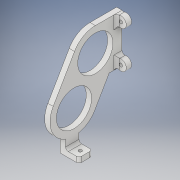
# Autodesk Inventor part: Tank Mount
Saved by Autodesk Inventor 2019.4 (Build 234330000, 330)
## iProperties
Created: 2020-01-30
Part Number: Tank Mount
Material: ABS Plastic
Document SubType Name: Modeling
Designer: admin
Mass: 80 g
Surface Area: 347.05 cm^2
Volume: 116.718 cm^3
Density: 0.685414 g/cm^3
Appearance: Smooth - White
Author: admin
Autodesk Inventor part; units mm, degrees
ref_plane "YZ Plane" through (0, 0, 0) normal (1, 0, 0) x (0, 1, 0)
ref_plane "XZ Plane" through (0, 0, 0) normal (0, 1, 0) x (-1, 0, 0)
ref_plane "XY Plane" through (0, 0, 0) normal (0, 0, 1) x (1, 0, 0)
sketch "Sketch1" plane through (0, 0, 0) normal (1, 0, 0) x (0, 1, 0)
  circle A0 centre (0, 0) radius 33
  circle A1 centre (69.282, -40) radius 33
  line L0 (0, 0) -> (69.282, -40) construction
  line L1 (69.282, -40) -> (69.282, -90) construction
  arc A2 (91.782, -1.0289) -> (114.282, -40) centre (69.282, -40) ccw construction
  arc A3 (-42.1724, 15.7) -> (-44.0285, -9.3) centre (0, 0) ccw construction
  line L2 (22.5, 38.9711) -> (91.782, -1.0289)
  line L3 (46.782, -78.9711) -> (24.282, -65.9808) construction
  line L4 (114.282, -40) -> (114.282, -90)
  line L5 (114.282, -90) -> (24.282, -90)
  line L6 (24.282, -90) -> (24.282, -65.9808)
  arc A4 (114.282, -40) -> (91.782, -1.0289) centre (69.282, -40) ccw
  line L7 (-70, 15.7) -> (-70, -9.3)
  line L8 (-70, 15.7) -> (-42.1724, 15.7)
  line L9 (-70, -9.3) -> (-44.0285, -9.3)
  arc A5 (22.5, 38.9711) -> (-42.1724, 15.7) centre (0, 0) ccw
  line L10 (24.282, -65.9808) -> (24.282, -40) construction
  line L11 (24.282, -65.9808) -> (-22.5, -38.9711)
  arc A6 (-22.5, -38.9711) -> (22.5, 38.9711) centre (0, 0) ccw construction
  arc A7 (-44.0285, -9.3) -> (-22.5, -38.9711) centre (0, 0) ccw
  dimension "d0" = 66
  dimension "d1" = 66
  dimension "d2" = 80
  dimension "d3" = 50
  dimension "d4" = 90
  dimension "d5" = 90
  dimension "d6" = 90
  dimension "d7" = 50
  dimension "d8" = 25
  dimension "d9" = 70
  dimension "d10" = 105.7
  constraints: 24 end point, 15 point on circle, 13 tangent, 8 centre point, 3 coincident, 3 parallel, 3 perpendicular, 3 vertical, 1 horizontal
  measures "d0" diameter of A0
  measures "d1" diameter of A1
  measures "d2" distance of L0.start L0.end
  measures "d3" distance of L0.end L1.end
  measures "d4" vertical distance of L1.end L0.start
  measures "d5" diameter of A2
  measures "d6" diameter of A3
  measures "d7" distance of L4.start L4.end
  measures "d8" distance of L7.start L7.end
  measures "d9" distance from line of point (0, 0) L7
  measures "d10" distance between parallel lines of L5 L8
extrude "Extrusion1" add sketch "Sketch1" along normal blind 10
sketch "Sketch2" plane through (0, -70, -9.3) normal (0, -1, 0) x (1, 0, 0)
  line L0 (0, 25) -> (35, 25)
  line L1 (35, 25) -> (35, 0)
  line L2 (35, 0) -> (0, 0)
  line L3 (0, 0) -> (0, 25)
  line L4 (0, 0) -> (0, 25) projected
  line L5 (0, 0) -> (10, 0) projected
  line L6 (10, 25) -> (10, 0) projected
  line L7 (0, 25) -> (10, 25) projected
  line L8 (0, 25) -> (10, 25) projected
  circle A0 centre (25, 12.5) radius 3
  line L9 (0, 48.2711) -> (0, 8.2711) projected
  point P0 (0, 9.3)
  dimension "d13" = 6
  dimension "d17" = 10
  dimension "d31" = 25
  constraints: 8 end point, 3 collinear, 2 parallel, 1 centre point, 1 horizontal, 1 perpendicular
  measures "d13" diameter of A0
  measures "d17" distance from line of L1 A0.centre
  measures "d31" distance between parallel lines of L6 L1
extrude "Extrusion2" add sketch "Sketch2" against normal blind 10 contours L0 L1 L2 L6
sketch "Sketch3" plane through (0, 24.282, -90) normal (0, 0, -1) x (-1, 0, 0)
  circle A0 centre (-18, 80) radius 3
  circle A1 centre (-18, 80) radius 10
  circle A2 centre (-18, 10) radius 3
  circle A3 centre (-18, 10) radius 10
  line L0 (0, 0) -> (-10, 0) projected
  line L1 (0, 90) -> (-10, 90) projected
  line L2 (0, 90) -> (0, 0) projected
  point P0 (0, -24.282)
  dimension "d23" = 6
  dimension "d24" = 20
  dimension "d25" = 6
  dimension "d26" = 20
  dimension "d32" = 18
  dimension "d33" = 18
  dimension "d36" = 10
  dimension "d37" = 10
  constraints: 4 centre point, 2 coincident
  measures "d23" diameter of A0
  measures "d24" diameter of A1
  measures "d25" diameter of A2
  measures "d26" diameter of A3
  measures "d32" distance from line of L2 A1.centre
  measures "d33" distance from line of L2 A3.centre
  measures "d36" distance from line of L1 A1.centre
  measures "d37" distance from line of L0 A3.centre
extrude "Extrusion3" add sketch "Sketch3" against normal blind 10
fillet "Fillet1" radius 5 3 edges at (35, -65, 15.7) (35, -65, -9.3) (10, -60, 3.2)
fillet "Fillet2" radius 5 5 edges at (10, 104.282, -80) (10, 34.282, -80) (10, 40.282, -85) (10, 98.282, -85) (10, 110.282, -85)
fillet "Fillet3" radius 1.5 1 edges at (10, 28.282, -82.5)
body "Solid1"
